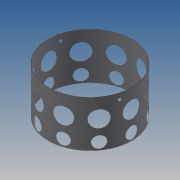
# Autodesk Inventor part: 2h1sin
Saved by Autodesk Inventor 2014 SP1 (Build 180222100, 222)
## iProperties
Company: HERA Project
Created: 2013-05-14
Part Number: 2h1sin
Material: Generic
Document SubType Name: Modeling
Designer: David DeBoer
Density: 1 g/cm^3
Description: Hub inner sonotube
Mass: 1625.04 g
Surface Area: 5665.19 cm^2
Volume: 1625.04 cm^3
Appearance: Default
Author: David DeBoer
Title: Hub innersono
Autodesk Inventor part; units mm, degrees
ref_plane "YZ Plane" through (0, 0, 0) normal (1, 0, 0) x (0, 1, 0)
ref_plane "XZ Plane" through (0, 0, 0) normal (0, 1, 0) x (-1, 0, 0)
ref_plane "XY Plane" through (0, 0, 0) normal (0, 0, 1) x (1, 0, 0)
sketch "Sketch1" plane through (0, 0, 0) normal (0, 1, 0) x (-1, 0, 0)
  circle A0 centre (0, 0) radius 230.124
  circle A1 centre (0, 0) radius 228.6
  dimension "d2" = 1.524
  dimension "d112" = 457.2
  constraints: 2 centre point, 1 coincident
  measures "d2" radial gap between concentric circles of A1 A0
  measures "d112" diameter of A1
extrude "tube" add sketch "Sketch1" along normal blind 254
sketch "Sketch2" plane through (0, 254, 0) normal (0, 1, 0) x (1, 0, 0)
  circle A0 centre (0, 0) radius 228.6 projected
  circle A1 centre (0, 0) radius 230.124 projected
  point P0 (-230.124, 0)
  constraints: 1 horizontal alignment, 1 other
ref_plane "Work Plane1" through (-230.124, 254, 0) normal (-1, 0, 0) x (0, -1, 0)
sketch "Sketch7" plane through (0, 254, 0) normal (0, 1, 0) x (1, 0, 0)
  circle A0 centre (0, 0) radius 228.6 projected
  circle A1 centre (0, 0) radius 230.124 projected
  line L0 (0, 0) -> (297.2113, -59.119) construction
  line L1 (0, 0) -> (303.0341, 0) construction
  point P0 (225.7022, -44.895)
  dimension "d45" = 11.25
  constraints: 4 end point, 1 equal length, 1 horizontal, 1 point on line, 2 other
  measures "d45" angle of L0 L1
ref_plane "Work Plane2" through (225.7022, 254, 44.895) normal (0.9807853, 0, 0.1950903) x (0, 1, 0)
sketch "Sketch15" plane through (0, 254, 0) normal (0, 1, 0) x (1, 0, 0)
  circle A0 centre (0, 0) radius 228.6 projected
  circle A1 centre (0, 0) radius 230.124 projected
  point P0 (-215.5686, -80.5434)
  constraints: 2 other
ref_plane "Work Plane5" through (-215.5686, 254, 80.5434) normal (-0.9367497, 0, 0.35) x (0, -1, 0)
sketch "Sketch17" plane through (0, 254, 0) normal (0, 1, 0) x (1, 0, 0)
  circle A0 centre (0, 0) radius 228.6 projected
  circle A1 centre (0, 0) radius 230.124 projected
  line L0 (0, 0) -> (-222.2827, 59.5605) construction
  line L1 (0, 0) -> (301.4465, 0) construction
  dimension "d97" = 165
  constraints: 4 end point, 1 coincident, 1 horizontal, 2 other
  measures "d97" angle of L1 L0
ref_plane "Work Plane7" through (-222.2827, 254, -59.5605) normal (-0.9659258, 0, -0.258819) x (0, -1, 0)
sketch "Sketch22" plane through (-222.2827, 254, -59.5605) normal (-0.9659258, 0, -0.258819) x (0, -1, 0)
  circle A0 centre (32, 0) radius 7.5
  line L0 (0, 230.124) -> (0, -230.124) projected
  point P0 (254, 0)
  dimension "d114" = 15
  dimension "d115" = 32
  constraints: 1 centre point
  measures "d114" diameter of A0
  measures "d115" distance from line of A0.centre L0
hole "rebar" at (-222.2827, 222, -59.5605) direction (0.9659258, 0, 0.258819) diameter 15 end through all
sketch "Sketch23" plane through (-230.124, 254, 0) normal (-1, 0, 0) x (0, -1, 0)
  line L0 (0.6055, -52.1695) -> (254, -52.1695)
  line L1 (254, -52.1695) -> (254, 52.1695)
  line L2 (254, 52.1695) -> (0.6055, 52.1695)
  line L3 (0.6055, 52.1695) -> (0.6055, -52.1695)
  point P0 (254, 0)
  constraints: 8 end point, 2 parallel, 1 horizontal, 1 perpendicular
extrude "fakeExtrude" add sketch "Sketch23" against normal blind 1
sketch "Sketch24" plane through (-230.124, 254, 0) normal (-1, 0, 0) x (0, 0, 1)
  line L0 (-52.1695, -254) -> (52.1695, -254) projected
  circle A0 centre (0, -214) radius 32
  circle A1 centre (0, -104) radius 45.5
  point P0 (0, -254)
  dimension "d126" = 91
  dimension "d127" = 64
  dimension "d128" = 40
  dimension "d129" = 150
  constraints: 2 centre point
  measures "d126" diameter of A1
  measures "d127" diameter of A0
  measures "d128" distance from line of L0 A0.centre
  measures "d129" distance from line of L0 A1.centre
extrude "sleeveSupportHoles" cut sketch "Sketch24" against normal through all
pattern_circular "Circular Pattern4" count 6 over 180 about axis through (0, 0, 0) along (0, 1, 0) of "sleeveSupportHoles"
body "Solid1"
